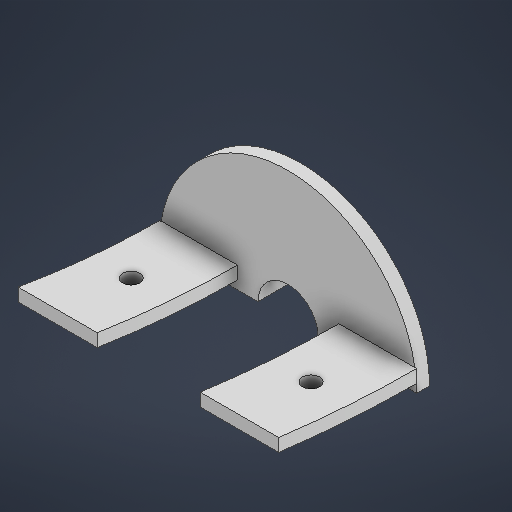
# Autodesk Inventor part: Verbindungsstück-links-15mm-Ph-L
Saved by Autodesk Inventor 2026.1 (Build 301233000, 233)
## iProperties
Created: 2025-11-03
Part Number: Verbindungsstück-links-15mm-Ph-L
Material: Generisch
Document SubType Name: Modeling
Designer: rebsa
Density: 1 g/cm^3
Appearance: Vorgabe
Author: rebsa
Autodesk Inventor part; units mm, degrees
ref_plane "YZ Plane" through (0, 0, 0) normal (1, 0, 0) x (0, 1, 0)
ref_plane "XZ Plane" through (0, 0, 0) normal (0, 1, 0) x (-1, 0, 0)
ref_plane "XY Plane" through (0, 0, 0) normal (0, 0, 1) x (1, 0, 0)
sketch "Skizze1" plane through (0, 0, 0) normal (0, 1, 0) x (-1, 0, 0)
  circle A0 centre (0, 0) radius 30
  circle A1 centre (0, 0) radius 7
  line L0 (7, 0) -> (30, 0)
  line L1 (-7, 0) -> (-30, 0)
  line L2 (42, 0) -> (-42, 0) projected
  line L3 (0, -42) -> (0, 42) projected
  dimension "d0" = 60
  dimension "d1" = 14
  dimension "d2" = 0
  constraints: 4 end point, 4 point on circle, 2 centre point, 2 point on line, 1 coincident, 1 concentric, 1 horizontal
  measures "d0" diameter of A0
  measures "d1" diameter of A1
  measures "d2" distance between parallel lines of L2 L1
extrude "Extrusion1" add sketch "Skizze1" along normal blind 3 contours L0 A1 L3 A0 | L3 A1 L1 A0 picked at (15.508, 15.8775) picked at (-21.0338, 7.0833)
sketch "Skizze3" plane through (0, 3, 0) normal (0, 1, 0) x (1, 0, 0)
  circle A0 centre (0, 0) radius 7.9
  circle A1 centre (0, 0) radius 7
  arc A2 (-7, 0) -> (7, 0) centre (0, 0) ccw projected
  line L0 (30, 0) -> (7, 0) projected
  line L1 (7.9, 0) -> (-7.9, 0)
  dimension "d13" = 15.8
  constraints: 2 centre point, 2 concentric, 2 end point, 2 point on circle, 1 coincident, 1 collinear, 1 point on line
  measures "d13" diameter of A0
extrude "Extrusion3" add sketch "Skizze3" along normal blind 15 contours A0 L1 A1 L0 picked at (7.5235, -0.6302)
sketch "Skizze7" plane through (-7, 0, 0) normal (0, 0, -1) x (-1, 0, 0)
  line L0 (466.8404, 0) -> (-120.9734, 0) projected
  line L1 (-7, -293.9069) -> (-7, 293.9069) projected
  line L2 (-37, 0) -> (-37, 3) projected
  circle A0 centre (172.9335, 0) radius 209.9335
  circle A1 centre (172.9335, 0) radius 191.832
  circle A2 centre (172.9335, 0) radius 168.168
  circle A3 centre (172.9335, 0) radius 150.0665
  line L3 (25.8962, -30) -> (-34.8454, -30)
  line L4 (0, 0) -> (23, 0) projected
  point P0 (-7, 0)
  point P1 (11.5, 0)
  point P2 (-16.5382, -30)
  point P3 (-18.8985, 0)
  point P4 (7.463, -30)
  point P5 (22.867, 0)
  point P6 (4.7655, 0)
  dimension "d45" = 419.867
  dimension "d48" = 300.133
  dimension "d46" = 383.664
  dimension "d47" = 336.336
  dimension "d49" = 30
  constraints: 2 centre point, 2 end point, 2 midpoint, 1 coincident, 1 concentric, 1 horizontal, 1 vertical, 7 other
  measures "d46" diameter of A1
  measures "d47" diameter of A2
  measures "d49" distance from line of point (11.5, 0) L3
extrude "Extrusion6" add sketch "Skizze7" against normal blind 5 contours L0 A1 L3 A0 | L0 A3 L3 A2 picked at (19.1917, -26.6918)
sketch "Skizze8" plane through (-30, 0, 0) normal (0, 0, -1) x (-1, 0, 0)
  circle A0 centre (149.9335, 0) radius 209.9335
  circle A1 centre (149.9335, 0) radius 191.832
  circle A2 centre (149.9335, 0) radius 168.168
  circle A3 centre (149.9335, 0) radius 150.0665
  arc A4 (-60, 0) -> (-57.8454, -30) centre (149.9335, 0) ccw projected
  line L0 (2.8962, -30) -> (-15.537, -30) projected
  line L1 (2.8962, -30) -> (-57.8454, -30)
  line L2 (-0.4196, 0) -> (-18.2345, 0) projected
  line L3 (-0.4196, 0) -> (-60, 0)
  line L4 (-0.4196, 0) -> (-59.5804, 0) projected
  line L5 (-0.4196, 0) -> (-0.133, 0)
  point P0 (-30, 0)
  point P1 (-211.1665, -40.8606)
  point P2 (-213.5268, -10.8606)
  point P3 (-231.6283, -10.8606)
  point P4 (-187.1653, -40.8606)
  point P5 (-171.7613, -10.8606)
  point P6 (-189.8628, -10.8606)
  point P7 (-41.8985, 0)
  point P8 (-57.8454, -30)
  point P9 (-39.5382, -30)
  dimension "d52" = 419.867
  dimension "d53" = 383.664
  dimension "d54" = 336.336
  dimension "d55" = 300.133
  constraints: 6 end point, 4 centre point, 3 concentric, 2 collinear, 1 coincident, 1 point on circle, 1 point on line
  measures "d52" diameter of A0
  measures "d53" diameter of A1
  measures "d54" diameter of A2
  measures "d55" diameter of A3
extrude "Extrusion7" cut sketch "Skizze8" against normal blind 2 contours L3 A1 L1 A0 | A2 L2 L5 A3 L0 picked at (-46.0773, -26.6819) picked at (-3.8083, -26.6918)
sketch "Skizze9" plane through (-7, 0, 5) normal (0, 0, 1) x (1, 0, 0)
  circle A0 centre (-172.9335, 0) radius 200.8827
  line L0 (-456.0871, 0) -> (119.8088, 0) projected
  line L1 (7, -281.2359) -> (7, 281.2359) projected
  arc A1 (34.8454, -30) -> (37, 0) centre (-172.9335, 0) ccw projected
  circle A2 centre (-172.9335, 0) radius 159.1173
  point P0 (7, 0)
  point P1 (-14.5249, -15)
  point P2 (27.3884, -15)
  dimension "d59" = 401.7655
  dimension "d60" = 318.2345
  dimension "d61" = 15
  dimension "d62" = 15
  constraints: 1 point on line, 7 other
  measures "d61" distance from line of point (27.388, -15) L0
  measures "d62" distance from line of L0 point (-14.525, -15)
hole "Bohrung2" at (-21.5249, -15, 5) at (20.3884, -15, 5) direction (0, 0, -1) diameter 4 depth 10 tip angle 118
